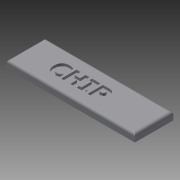
# Autodesk Inventor part: CHIP
Saved by Autodesk Inventor 2013 (Build 170138000, 138)
## iProperties
Created: 2014-07-07
Part Number: CHIP
Material: Genérico
Document SubType Name: Chapa
Designer: Administrador
Density: 1 g/cm^3
Sheet Metal Rule: Por defecto_mm
Author: Administrador
Autodesk Inventor part; units mm, degrees
note: some values were not read from the file. Chosen so that the rebuilt part matches the saved one: direction of "Repujado1".
ref_plane "YZ Plane" through (0, 0, 0) normal (1, 0, 0) x (0, 1, 0)
ref_plane "XZ Plane" through (0, 0, 0) normal (0, 1, 0) x (-1, 0, 0)
ref_plane "XY Plane" through (0, 0, 0) normal (0, 0, 1) x (1, 0, 0)
sketch "Boceto1" plane through (0, 0, 0) normal (0, 0, 1) x (1, 0, 0)
  line L0 (-8.6661, 3.3458) -> (41.3339, 3.3458)
  line L1 (41.3339, 3.3458) -> (41.3339, -11.6542)
  line L2 (41.3339, -11.6542) -> (-8.6661, -11.6542)
  line L3 (-8.6661, -11.6542) -> (-8.6661, 3.3458)
  point P0 (0, 0)
  dimension "d0" = 50
  dimension "d1" = 15
  constraints: 8 end point, 2 parallel, 1 horizontal, 1 perpendicular
  measures "d0" distance of L1.end L2.end
  measures "d1" distance of L0.end L1.end
extrude "Extrusión1" add sketch "Boceto1" along normal blind 3
sketch "Boceto2" plane through (0, 0, 3) normal (0, 0, 1) x (1, 0, 0)
  line L0 (2.2378, -1.3021) -> (23.4614, -1.3021) construction
  line L1 (23.4614, -1.3021) -> (23.4614, -7.5355) construction
  line L2 (23.4614, -7.5355) -> (2.2378, -7.5355) construction
  line L3 (2.2378, -7.5355) -> (2.2378, -1.3021) construction
  spline S0 degree 2 poles (5.4469, -7.5355) (4.0952, -7.5355) (2.5101, -5.9018) (2.5101, -4.4237) knots 0 0 0 1 2 2 2
  spline S1 degree 2 poles (2.5101, -4.4237) (2.5101, -2.999) (4.1, -1.3021) (5.4517, -1.3021) knots 0 0 0 1 2 2 2
  spline S2 degree 2 poles (5.4517, -1.3021) (5.8067, -1.3021) (6.3804, -1.3848) (6.643, -1.4528) knots 0 0 0 1 2 2 2
  spline S3 degree 2 poles (6.643, -1.4528) (6.8472, -1.516) (7.3285, -1.7251) (7.4793, -1.8029) knots 0 0 0 1 2 2 2
  line L4 (7.4793, -1.8029) -> (7.4793, -3.2324)
  line L5 (7.4793, -3.2324) -> (7.3285, -3.2324)
  spline S4 degree 2 poles (7.3285, -3.2324) (7.2167, -3.1352) (6.8861, -2.8629) (6.677, -2.7365) knots 0 0 0 1 2 2 2
  spline S5 degree 2 poles (6.677, -2.7365) (6.4679, -2.6052) (5.9671, -2.4253) (5.69, -2.4253) knots 0 0 0 1 2 2 2
  spline S6 degree 2 poles (5.69, -2.4253) (5.3642, -2.4253) (4.8245, -2.6295) (4.5765, -2.8872) knots 0 0 0 1 2 2 2
  spline S7 degree 2 poles (4.5765, -2.8872) (4.3529, -3.1157) (4.066, -3.8985) (4.066, -4.4285) knots 0 0 0 1 2 2 2
  spline S8 degree 2 poles (4.066, -4.4285) (4.066, -4.9877) (4.3626, -5.751) (4.6057, -5.9844) knots 0 0 0 1 2 2 2
  spline S9 degree 2 poles (4.6057, -5.9844) (4.8391, -6.213) (5.4128, -6.4123) (5.6997, -6.4123) knots 0 0 0 1 2 2 2
  spline S10 degree 2 poles (5.6997, -6.4123) (5.9963, -6.4123) (6.536, -6.213) (6.7208, -6.0914) knots 0 0 0 1 2 2 2
  spline S11 degree 2 poles (6.7208, -6.0914) (6.925, -5.9698) (7.2313, -5.7121) (7.3431, -5.61) knots 0 0 0 1 2 2 2
  line L6 (7.3431, -5.61) -> (7.4793, -5.61)
  line L7 (7.4793, -5.61) -> (7.4793, -7.0201)
  spline S12 degree 2 poles (7.4793, -7.0201) (7.314, -7.0979) (6.8812, -7.2924) (6.6478, -7.3604) knots 0 0 0 1 2 2 2
  spline S13 degree 2 poles (6.6478, -7.3604) (6.3658, -7.448) (5.8747, -7.5355) (5.4469, -7.5355) knots 0 0 0 1 2 2 2
  line L8 (13.4307, -7.4188) -> (11.9234, -7.4188)
  line L9 (11.9234, -7.4188) -> (11.9234, -4.7591)
  line L10 (11.9234, -4.7591) -> (9.8764, -4.7591)
  line L11 (9.8764, -4.7591) -> (9.8764, -7.4188)
  line L12 (9.8764, -7.4188) -> (8.3691, -7.4188)
  line L13 (8.3691, -7.4188) -> (8.3691, -1.4188)
  line L14 (8.3691, -1.4188) -> (9.8764, -1.4188)
  line L15 (9.8764, -1.4188) -> (9.8764, -3.6165)
  line L16 (9.8764, -3.6165) -> (11.9234, -3.6165)
  line L17 (11.9234, -3.6165) -> (11.9234, -1.4188)
  line L18 (11.9234, -1.4188) -> (13.4307, -1.4188)
  line L19 (13.4307, -1.4188) -> (13.4307, -7.4188)
  line L20 (17.6608, -7.4188) -> (14.4323, -7.4188)
  line L21 (14.4323, -7.4188) -> (14.4323, -6.3734)
  line L22 (14.4323, -6.3734) -> (15.2929, -6.3734)
  line L23 (15.2929, -6.3734) -> (15.2929, -2.4642)
  line L24 (15.2929, -2.4642) -> (14.4323, -2.4642)
  line L25 (14.4323, -2.4642) -> (14.4323, -1.4188)
  line L26 (14.4323, -1.4188) -> (17.6608, -1.4188)
  line L27 (17.6608, -1.4188) -> (17.6608, -2.4642)
  line L28 (17.6608, -2.4642) -> (16.8002, -2.4642)
  line L29 (16.8002, -2.4642) -> (16.8002, -6.3734)
  line L30 (16.8002, -6.3734) -> (17.6608, -6.3734)
  line L31 (17.6608, -6.3734) -> (17.6608, -7.4188)
  spline S14 degree 2 poles (23.2767, -3.3102) (23.2767, -3.7284) (23.0093, -4.4869) (22.7613, -4.7397) knots 0 0 0 1 2 2 2
  spline S15 degree 2 poles (22.7613, -4.7397) (22.6106, -4.9002) (22.241, -5.1627) (22.0222, -5.2551) knots 0 0 0 1 2 2 2
  spline S16 degree 2 poles (22.0222, -5.2551) (21.7986, -5.3475) (21.2783, -5.4544) (20.9574, -5.4544) knots 0 0 0 1 2 2 2
  line L32 (20.9574, -5.4544) -> (20.1697, -5.4544)
  line L33 (20.1697, -5.4544) -> (20.1697, -7.4188)
  line L34 (20.1697, -7.4188) -> (18.6624, -7.4188)
  line L35 (18.6624, -7.4188) -> (18.6624, -1.4188)
  line L36 (18.6624, -1.4188) -> (20.9914, -1.4188)
  spline S17 degree 2 poles (20.9914, -1.4188) (21.5068, -1.4188) (22.2605, -1.6084) (22.5668, -1.8126) knots 0 0 0 1 2 2 2
  spline S18 degree 2 poles (22.5668, -1.8126) (22.9072, -2.0412) (23.2767, -2.7899) (23.2767, -3.3102) knots 0 0 0 1 2 2 2
  spline S19 degree 2 poles (21.7305, -3.3491) (21.7305, -3.0914) (21.4874, -2.7267) (21.3221, -2.6587) knots 0 0 0 1 2 2 2
  spline S20 degree 2 poles (21.3221, -2.6587) (21.1081, -2.5663) (20.7191, -2.5371) (20.3837, -2.5371) knots 0 0 0 1 2 2 2
  line L37 (20.3837, -2.5371) -> (20.1697, -2.5371)
  line L38 (20.1697, -2.5371) -> (20.1697, -4.3361)
  line L39 (20.1697, -4.3361) -> (20.2767, -4.3361)
  spline S21 degree 2 poles (20.2767, -4.3361) (20.4858, -4.3361) (20.865, -4.3264) (21.006, -4.3021) knots 0 0 0 1 2 2 2
  spline S22 degree 2 poles (21.006, -4.3021) (21.1276, -4.2826) (21.395, -4.166) (21.4679, -4.093) knots 0 0 0 1 2 2 2
  spline S23 degree 2 poles (21.4679, -4.093) (21.6235, -3.9472) (21.7305, -3.6214) (21.7305, -3.3491) knots 0 0 0 1 2 2 2
  point P0 (0, 0)
  constraints: 2 other
emboss "Repujado1" sketch "Boceto2" operation cut depth 1 direction (0, 0, -1)
fillet "Empalme1" radius 1 4 edges at (16.3339, 3.3458, 3) (41.3339, -4.1542, 3) (-8.6661, -4.1542, 3) (16.3339, -11.6542, 3)
equation "\"Radio_pliegue\" = Grosor"
equation "\"Anchura_desahogo_plegado\" = Grosor"
equation "\"Profundidad_desahogo_plegado\" = 0.5 * Grosor"
equation "\"Tamaño_destalonado\" = 4 * Grosor"
equation "\"Remanente_mínimo\" = 2 * Grosor"
equation "\"Radiodetransición\" = Radio_pliegue"
equation "\"Tamaño_de_radio_de_Jacobi\" = Radio_pliegue"
equation "\"TamañoSeparación\" = Grosor"
equation "\"Grosor\" = 0.5"
